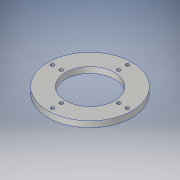
# Autodesk Inventor part: Bearing
Saved by Autodesk Inventor 2019.4 (Build 234330000, 330)
## iProperties
Created: 2019-11-30
Part Number: Bearing
Material: Aluminum 6061
Document SubType Name: Modeling
Designer: admin
Density: 2.96364 g/cm^3
Appearance: Aluminum - Flat
Mass: 184 g
Surface Area: 207.502 cm^2
Volume: 62.0857 cm^3
Author: admin
Autodesk Inventor part; units mm, degrees
ref_plane "YZ Plane" through (0, 0, 0) normal (1, 0, 0) x (0, 1, 0)
ref_plane "XZ Plane" through (0, 0, 0) normal (0, 1, 0) x (-1, 0, 0)
ref_plane "XY Plane" through (0, 0, 0) normal (0, 0, 1) x (1, 0, 0)
sketch "Sketch1" plane through (0, 0, 0) normal (0, 1, 0) x (-1, 0, 0)
  circle A0 centre (0, 0) radius 35
  circle A1 centre (0, 0) radius 60
  dimension "d0" = 70
  dimension "d1" = 120
  constraints: 2 centre point, 2 coincident
  measures "d0" diameter of A0
  measures "d1" diameter of A1
extrude "Extrusion1" add sketch "Sketch1" along normal blind 8.5
sketch "Sketch2" plane through (0, 8.5, 0) normal (0, 1, 0) x (1, 0, 0)
  circle A0 centre (-41, 0) radius 2.5
  circle A1 centre (-53.5, 0) radius 2.5
  line L0 (-41, 0) -> (0, 0) construction
  line L1 (-41, 0) -> (-53.5, 0) construction
  dimension "d4" = 5
  dimension "d5" = 5
  dimension "d6" = 41
  dimension "d7" = 53.5
  constraints: 4 end point, 2 centre point, 2 horizontal
  measures "d4" diameter of A0
  measures "d5" diameter of A1
  measures "d6" distance of L0.start L0.end
  measures "d7" distance of L0.end L1.end
extrude "Extrusion2" cut sketch "Sketch2" against normal through all
pattern_circular "Circular Pattern1" count 4 over 360 about axis through (0, 0, 0) along (0, 1, 0) of "Extrusion2"
body "Solid1"
